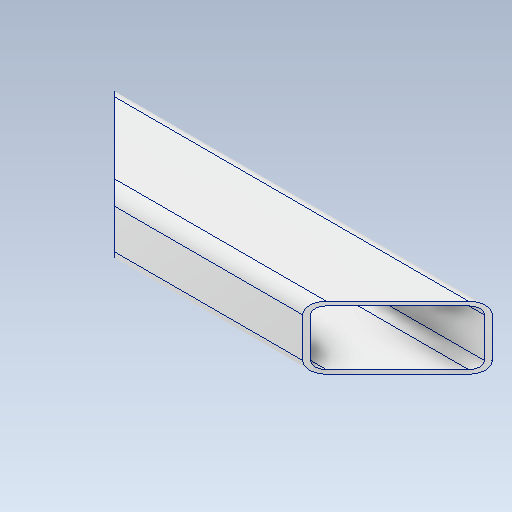
# Autodesk Inventor part: back bar
Saved by Autodesk Inventor 2021 (Build 250183000, 183)
## iProperties
Created: 2021-03-29
Part Number: back bar
Material: Aluminum 6061
Document SubType Name: Modeling
Designer: Work
Mass: 444.213 g
Surface Area: 1056.81 cm^2
Volume: 164.523 cm^3
Density: 2.7 g/cm^3
Appearance: Aluminum - Flat
Author: Work
Autodesk Inventor part; units mm, degrees
ref_plane "YZ Plane" through (0, 0, 0) normal (1, 0, 0) x (0, 1, 0)
ref_plane "XZ Plane" through (0, 0, 0) normal (0, 1, 0) x (-1, 0, 0)
ref_plane "XY Plane" through (0, 0, 0) normal (0, 0, 1) x (1, 0, 0)
sketch "Sketch1" plane through (0, 0, 0) normal (1, 0, 0) x (0, 1, 0)
  line L0 (-15.875, 38.1) -> (15.875, 38.1)
  line L1 (25.4, 28.575) -> (25.4, -28.575)
  line L2 (15.875, -38.1) -> (-15.875, -38.1)
  line L3 (-25.4, -28.575) -> (-25.4, 28.575)
  line L4 (-25.4, 38.1) -> (25.4, -38.1) construction
  line L5 (25.4, 38.1) -> (-25.4, -38.1) construction
  arc A0 (25.4, 28.575) -> (15.875, 38.1) centre (15.875, 28.575) ccw
  arc A1 (-15.875, 38.1) -> (-25.4, 28.575) centre (-15.875, 28.575) ccw
  arc A2 (-25.4, -28.575) -> (-15.875, -38.1) centre (-15.875, -28.575) ccw
  arc A3 (15.875, -38.1) -> (25.4, -28.575) centre (15.875, -28.575) ccw
  line L6 (22.225, -28.575) -> (22.225, 28.575)
  arc A4 (22.225, 28.575) -> (15.875, 34.925) centre (15.875, 28.575) ccw
  line L7 (15.875, 34.925) -> (-15.875, 34.925)
  arc A5 (-15.875, 34.925) -> (-22.225, 28.575) centre (-15.875, 28.575) ccw
  line L8 (-22.225, 28.575) -> (-22.225, -28.575)
  arc A6 (-22.225, -28.575) -> (-15.875, -34.925) centre (-15.875, -28.575) ccw
  line L9 (-15.875, -34.925) -> (15.875, -34.925)
  arc A7 (15.875, -34.925) -> (22.225, -28.575) centre (15.875, -28.575) ccw
  point P0 (0, 0)
  dimension "d0" = 76.2
  dimension "d1" = 50.8
  dimension "d2" = 9.525
  dimension "d3" = 3.175
  constraints: 20 end point, 16 point on circle, 8 centre point, 8 point on line, 8 tangent, 4 parallel, 3 equal radius, 2 midpoint, 2 perpendicular, 1 horizontal, 7 other
  measures "d0" distance of L5.start L4.end
  measures "d1" distance of L4.end L5.end
  measures "d2" radius of A0
  measures "d3" distance between parallel lines of L6 L1
extrude "Extrusion1" add sketch "Sketch1" along normal mid plane 303.8
sketch "Sketch2" plane through (-151.9, 25.4, 28.575) normal (0, 1, 0) x (1, 0, 0)
  line L0 (303.8, 57.15) -> (303.8, 66.675) projected
  line L1 (303.8, 66.675) -> (227.6, -9.525)
  line L2 (0, -9.525) -> (303.8, -9.525) projected
  line L3 (303.8, 66.675) -> (411.5631, 66.675) construction
  line L4 (227.6, -9.525) -> (303.8, -9.525)
  line L5 (303.8, -9.525) -> (303.8, 66.675)
  line L6 (151.9, 28.575) -> (151.9, -9.525)
  line L7 (0, 66.675) -> (76.2, -9.525)
  line L8 (76.2, -9.525) -> (0, -9.525)
  line L9 (0, -9.525) -> (0, 66.675)
  dimension "d6" = 135
  constraints: 16 end point, 2 point on line, 2 symmetric about line, 1 collinear, 1 equal length, 1 horizontal, 1 parallel, 1 perpendicular
  measures "d6" angle of L1 L3
extrude "Extrusion2" cut sketch "Sketch2" against normal through all
equation "\"d0\" = stockWidth"
equation "\"d1\" = stockHeight"
equation "\"d2\" = stockRad"
equation "\"d3\" = stockGuage"
equation "\"height\" = 203.2"
equation "\"shaftDiam\" = 6.35"
equation "\"shaftSpace\" = 1.5875"
equation "\"stageSpace\" = 2.54"
equation "\"stageAngle\" = 15deg"
equation "\"stockHeight\" = 50.8"
equation "\"stockWidth\" = 76.2"
equation "\"stockRad\" = 9.525"
equation "\"stockGuage\" = 3.175"
equation "\"groundActu\" = 304.8"
equation "\"baseWidth\" = 1066.8"
equation "\"baseDepth\" = 254"
equation "\"capThickness\" = 3.175"
equation "\"sup1Ang\" = 22.619865deg"
equation "\"sup1Len\" = 660.4"
equation "\"supVertLen\" = 955.13561"
equation "\"sup2Ang\" = 8.959949deg"
equation "\"sup2Len\" = 2079.37366"
equation "\"supSideAng\" = 19.376933deg"
equation "\"supSideLen\" = 1531.12879"
equation "\"FlangeDiam\" = 12.7"
equation "\"bearingDiam\" = 9.5504"
equation "\"FlangeDepth\" = 1.5875"
equation "\"smallFilet\" = 0.39687"
equation "\"thickness\" = 12.7"
equation "\"ringDiam\" = 96.46608"
body "Solid1"
